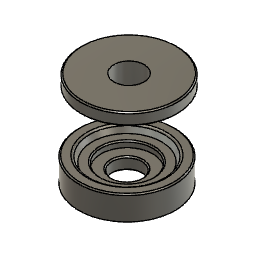
Drain_Dimple_Die_Mod2V1 (Autodesk Fusion 360 design; units mm, degrees)
Autodesk Fusion 360 part; units mm, degrees
sketch "Sketch1" plane through (0, 0, 0) normal (1, 0, 0) x (0, 0, -1)
  line L0 (7.9375, 0) -> (12.7, 0)
  line L1 (12.7, 0) -> (12.7, 3.175)
  line L2 (12.7, 3.175) -> (17.78, 3.175)
  line L3 (17.78, 3.175) -> (19.6131, 6.35)
  line L4 (19.6131, 6.35) -> (25.4, 6.35)
  line L5 (25.4, 6.35) -> (25.4, 12.7)
  line L6 (25.4, 12.7) -> (7.9375, 12.7)
  line L7 (7.9375, 0) -> (7.9375, 12.7)
  line L8 (7.9375, -1) -> (13.7, -1)
  line L9 (13.7, -1) -> (13.7, 2.175)
  line L10 (13.7, 2.175) -> (18.3574, 2.175)
  line L11 (18.3574, 2.175) -> (20.1904, 5.35)
  line L12 (20.1904, 5.35) -> (25.4, 5.35)
  line L13 (25.4, 5.35) -> (25.4, -7.35)
  line L14 (25.4, -7.35) -> (7.9375, -7.35)
  line L15 (7.9375, -7.35) -> (7.9375, -1)
  dimension "d2" = 3.175
  dimension "d3" = 5.08
  dimension "d4" = 60
  dimension "d5" = 6.35
  dimension "d9" = 12.7
  dimension "d10" = 7.9375
  dimension "d11" = 4.7625
  dimension "d12" = 17.4625
  dimension "d13" = 1
  dimension "d14" = 6.35
  dimension "d15" = 5.7625
  dimension "d16" = 3.175
  dimension "d17" = 4.6573
  dimension "d18" = 5.2096
  dimension "d19" = 12.7
  dimension "d20" = 3.175
  constraint horizontal L0
  constraint perpendicular L0 L1
  constraint perpendicular L1 L2
  constraint perpendicular L1 L4
  constraint perpendicular L4 L5
  constraint perpendicular L5 L6
  constraint perpendicular L6 L7
  constraint perpendicular L12 L13
  constraint perpendicular L13 L14
  constraint vertical L15
  measures "d2" distance of L0.end L1.end
  measures "d3" distance of L1.end L2.end
  measures "d4" angle of L2 L3
  measures "d5" distance of origin L4
  measures "d9" distance of L0.start L6.end
  measures "d10" distance of origin L7
  measures "d11" distance of L0.end L0.start
  measures "d12" distance of L5.end L6.end
  measures "d14" distance of L8.start L14.end
  measures "d15" distance of L8.start L8.end
  measures "d16" distance of L8.end L9.end
  measures "d17" distance of L9.end L10.end
  measures "d18" distance of L11.end L12.end
  measures "d19" distance of L12.end L13.end
  measures "d20" vertical distance of L2.end L3.end
revolve "Revolve1" add sketch "Sketch1" angle 360 about axis through (0, 1.75, 0) along (0, 1, 0) makes body 1 at (1.6562, 12.7, -19.455) makes body 2 at (2.529, 1.1167, -25.2738)
copy_body "Body->Comp1" bodies 2 removing the originals makes body 3 in component "Die"
copy_body "Body->Comp2" bodies 1 removing the originals makes body 4 in component "Punch"
chamfer "Chamfer1" distance 0.635 angle 45 2 edges at (-23.6811, 6.35, -9.185) (-23.6811, 12.7, -9.185) on bodies 4 in component "Punch"
chamfer "Chamfer2" distance 0.635 angle 45 1 edges at (-11.8406, 0, -4.5925) on bodies 4 in component "Punch"
chamfer "Chamfer1'" distance 0.635 angle 45 4 edges at (-23.6811, 5.35, -9.185) (-12.7729, 2.175, -4.9541) (-7.4003, -1, -2.8703) (-7.4003, -7.35, -2.8703) on bodies 3 in component "Die"
fillet "Fillet1" radius 1.27 1 edges at (-18.8241, 5.35, -7.3012) on bodies 3 in component "Die"
fillet "Fillet1'" radius 1.27 1 edges at (-16.5768, 3.175, -6.4295) on bodies 4 in component "Punch"
component "Die" placed x (1, 0, 0) y (0, 1, 0) z (0, 0, 1) at (-14.6517, -12.3125, 22.8626)
component "Punch" placed x (1, 0, 0) y (0, 1, 0) z (0, 0, 1) at (7.3379, 12.6646, -16.4943)
